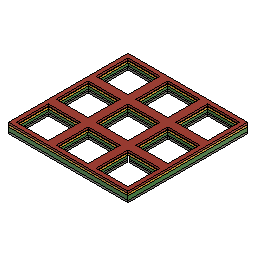
One Face (Autodesk Fusion 360 design; units mm, degrees)
Autodesk Fusion 360 part; units mm, degrees
note: some values were not read from the file. Set by a fixed rule: which sketch regions a step uses.
sketch "OldFirstLayer" plane through (0, 0, 0) normal (0, 0, 1) x (1, 0, 0)
  line L0 (-176.2126, -49.2126) -> (-176.2126, 49.2124)
  line L1 (-77.7876, 49.2124) -> (-77.7876, -49.2126)
  line L2 (-77.7876, 77.7874) -> (-176.2126, 77.7874)
  line L3 (-77.7876, 176.2124) -> (-77.7876, 77.7874)
  line L4 (-176.2126, 176.2124) -> (-77.7876, 176.2124)
  line L5 (-176.2126, -176.2126) -> (-176.2126, -77.7876)
  line L6 (-77.7876, -86.1838) -> (-77.7876, -176.2126)
  line L7 (-176.2126, 49.2124) -> (-77.7876, 49.2124)
  line L8 (-77.7876, -176.2126) -> (-176.2126, -176.2126)
  line L9 (49.2124, -82.6672) -> (49.2124, -176.2126)
  line L10 (190.4999, -190.5001) -> (190.4999, 190.4999)
  line L11 (49.2124, 176.2124) -> (49.2124, 77.7874)
  line L12 (176.2124, -176.2126) -> (77.7874, -176.2126)
  line L13 (77.7874, -49.2126) -> (77.7874, 49.2124)
  line L14 (176.2124, -49.2126) -> (77.7874, -49.2126)
  line L15 (77.7874, 49.2124) -> (170.2008, 49.2124)
  line L16 (176.2124, 176.2124) -> (176.2124, 77.7874)
  line L17 (176.2124, 49.2124) -> (176.2124, -49.2126)
  line L18 (49.2124, 49.2124) -> (49.2124, -49.2126)
  line L19 (77.7874, -77.7876) -> (176.2124, -77.7876)
  line L20 (77.7874, -176.2126) -> (77.7874, -82.6672)
  line L21 (77.7874, 176.2124) -> (176.2124, 176.2124)
  line L22 (170.2008, 77.7874) -> (77.7874, 77.7874)
  line L23 (176.2124, -77.7876) -> (176.2124, -176.2126)
  line L24 (77.7874, 77.7874) -> (77.7874, 176.2124)
  line L25 (-190.5001, 190.4999) -> (-190.5001, -190.5001)
  line L26 (-77.7876, -49.2126) -> (-176.2126, -49.2126)
  line L27 (190.4999, 190.4999) -> (-190.5001, 190.4999)
  line L28 (-49.2126, -77.7876) -> (49.2124, -77.7876)
  line L29 (-49.2126, -49.2126) -> (-49.2126, 49.2124)
  line L30 (49.2124, 77.7874) -> (-49.2126, 77.7874)
  line L31 (-49.2126, 176.2124) -> (49.2124, 176.2124)
  line L32 (-176.2126, -77.7876) -> (-77.7876, -77.7876)
  line L33 (-176.2126, 77.7874) -> (-176.2126, 176.2124)
  line L34 (-49.2126, -176.2126) -> (-49.2126, -86.1838)
  line L35 (-190.5001, -190.5001) -> (190.4999, -190.5001)
  line L36 (49.2124, -49.2126) -> (-49.2126, -49.2126)
  line L37 (49.2124, -176.2126) -> (-49.2126, -176.2126)
  line L38 (-49.2126, 77.7874) -> (-49.2126, 176.2124)
  line L39 (-190.5001, 190.4999) -> (190.4999, -190.5001) construction
  line L40 (-49.2126, 49.2124) -> (49.2124, 49.2124)
  line L41 (190.4999, 190.4999) -> (-190.5001, -190.5001) construction
  line L42 (170.2008, 77.7874) -> (170.2008, 49.2124)
  line L43 (176.2124, 77.7874) -> (176.2124, 49.2124)
  line L44 (49.2124, -82.6672) -> (77.7874, -82.6672)
  line L45 (49.2124, -77.7876) -> (77.7874, -77.7876)
  line L46 (-77.7876, -77.7876) -> (-49.2126, -77.7876)
  line L47 (-77.7876, -86.1838) -> (-77.7876, -83.82)
  line L48 (-49.2126, -86.1838) -> (-49.2126, -83.82)
  line L49 (-77.7876, -83.82) -> (-49.2126, -83.82)
  point P0 (-0.0001, -0.0001)
  point P1 (-0.0001, -0.0001)
  dimension "d57" = 381
  dimension "d58" = 381
  dimension "d59" = 98.425
  dimension "d60" = 98.425
  dimension "d61" = 28.575
  dimension "d62" = 98.425
  dimension "d63" = 98.425
  dimension "d64" = 28.575
  dimension "d65" = 98.425
  dimension "d66" = 98.425
  dimension "d67" = 28.575
  dimension "d68" = 98.425
  dimension "d69" = 98.425
  dimension "d70" = 98.425
  dimension "d71" = 98.425
  dimension "d72" = 28.575
  dimension "d73" = 98.425
  dimension "d74" = 98.425
  dimension "d75" = 28.575
  dimension "d76" = 28.575
  dimension "d77" = 98.425
  dimension "d78" = 98.425
  dimension "d80" = 28.575
  dimension "d81" = 98.425
  dimension "d82" = 98.425
  dimension "d83" = 98.425
  dimension "d84" = 98.425
  dimension "d85" = 28.575
  dimension "d86" = 28.575
  dimension "d87" = 28.575
  dimension "d88" = 28.575
  dimension "d89" = 14.2875
  dimension "d90" = 14.2875
  dimension "d91" = 14.2875
  dimension "d97" = 28.575
  dimension "d103" = 14.2875
  constraint perpendicular L25 L27
  constraint parallel L27 L35
  constraint parallel L10 L25
  constraint horizontal L27
  constraint coincident P1 L41
  constraint coincident P1 L39
  constraint coincident P1 P0
  constraint horizontal L4
  constraint vertical L3
  constraint horizontal L2
  constraint vertical L33
  constraint coincident L4.start L39
  constraint horizontal L7
  constraint vertical L1
  constraint horizontal L26
  constraint vertical L0
  constraint horizontal L32
  constraint vertical L6
  constraint horizontal L8
  constraint vertical L5
  constraint horizontal L31
  constraint vertical L11
  constraint horizontal L30
  constraint vertical L38
  constraint horizontal L21
  constraint vertical L16
  constraint horizontal L22
  constraint vertical L24
  constraint horizontal L40
  constraint vertical L18
  constraint horizontal L36
  constraint vertical L29
  constraint horizontal L15
  constraint vertical L17
  constraint horizontal L14
  constraint vertical L13
  constraint horizontal L19
  constraint vertical L23
  constraint horizontal L12
  constraint vertical L20
  constraint coincident L19.start L39
  constraint horizontal L28
  constraint vertical L9
  constraint horizontal L37
  constraint vertical L34
  constraint perpendicular L15 L42
  constraint perpendicular L20 L44
  constraint parallel L6 L47
  constraint perpendicular L46 L48
  constraint perpendicular L48 L49
  measures "d57" distance of L25.end L25.start
  measures "d58" distance of L10.end L25.start
  measures "d59" distance of L4.start L2.end
  measures "d60" distance of L4.start L3.start
  measures "d61" distance of L2 L7
  measures "d62" distance of L0.end L0.start
  measures "d63" distance of L0.end L1.start
  measures "d64" distance of L26 L32
  measures "d65" distance of L6.end L5.start
  measures "d66" distance of L6.end L32.end
  measures "d67" distance of L3 L38
  measures "d68" distance of L11.end L30.end
  measures "d69" distance of L11.end L11.start
  measures "d70" distance of L21.start L16.start
  measures "d71" distance of L16.start L16.end
  measures "d72" distance of L11 L24
  measures "d73" distance of L29.end L18.start
  measures "d74" distance of L29.end L29.start
  measures "d75" distance of L1 L29
  measures "d76" distance of L30 L40
  measures "d77" distance of L13.end L17.start
  measures "d78" distance of L13.start L13.end
  measures "d80" distance of L15 L22
  measures "d81" distance of L19.end L12.start
  measures "d82" distance of L19.start L19.end
  measures "d83" distance of L28.end L28.start
  measures "d84" distance of L34.start L28.start
  measures "d85" distance of L28 L36
  measures "d86" distance of L6 L34
  measures "d87" distance of L9 L20
  measures "d88" distance of L14 L19
  measures "d89" distance of L25 L33
  measures "d90" distance of L0 L25
  measures "d91" distance of L5 L25
  measures "d97" distance of L13 L18
  measures "d103" distance of L35 L37
sketch "ThirdLayerSketch" plane through (0, 0, 0) normal (0, 0, 1) x (1, 0, 0)
  line L0 (48.9649, -178.1983) -> (-49.4601, -178.1983)
  line L1 (-49.4601, 174.2267) -> (48.9649, 174.2267)
  line L2 (-49.4601, -79.7733) -> (48.9649, -79.7733)
  line L3 (48.9649, 47.2267) -> (48.9649, -51.1983)
  line L4 (48.9649, 174.2267) -> (48.9649, 75.8017)
  line L5 (77.5399, 174.2267) -> (175.9649, 174.2267)
  line L6 (175.9649, 174.2267) -> (175.9649, 75.8017)
  line L7 (175.9649, 47.2267) -> (175.9649, -51.1983)
  line L8 (-78.0351, -51.1983) -> (-176.4601, -51.1983)
  line L9 (175.9649, -178.1983) -> (77.5399, -178.1983)
  line L10 (48.9649, -79.7733) -> (48.9649, -178.1983)
  line L11 (175.9649, -51.1983) -> (77.5399, -51.1983)
  line L12 (-176.4601, -79.7733) -> (-78.0351, -79.7733)
  line L13 (-78.0351, -178.1983) -> (-176.4601, -178.1983)
  line L14 (175.9649, -79.7733) -> (175.9649, -178.1983)
  line L15 (77.5399, -178.1983) -> (77.5399, -79.7733)
  line L16 (77.5399, -79.7733) -> (175.9649, -79.7733)
  line L17 (-176.4601, 174.2267) -> (-78.0351, 174.2267)
  line L18 (-78.0351, 47.2267) -> (-78.0351, -51.1983)
  line L19 (-176.4601, 75.8017) -> (-176.4601, 174.2267)
  line L20 (-176.4601, -178.1983) -> (-176.4601, -79.7733)
  line L21 (77.5399, 47.2267) -> (175.9649, 47.2267)
  line L22 (77.5399, -51.1983) -> (77.5399, 47.2267)
  line L23 (-78.0351, -79.7733) -> (-78.0351, -178.1983)
  line L24 (175.9649, 75.8017) -> (77.5399, 75.8017)
  line L25 (-190.7476, 188.5142) -> (-190.7476, -192.4858)
  line L26 (190.2524, -192.4858) -> (190.2524, 188.5142)
  line L27 (77.5399, 75.8017) -> (77.5399, 174.2267)
  line L28 (-176.4601, -51.1983) -> (-176.4601, 47.2267)
  line L29 (-176.4601, 47.2267) -> (-78.0351, 47.2267)
  line L30 (-78.0351, 174.2267) -> (-78.0351, 75.8017)
  line L31 (-49.4601, 47.2267) -> (48.9649, 47.2267)
  line L32 (-78.0351, 75.8017) -> (-176.4601, 75.8017)
  line L33 (190.2524, 188.5142) -> (-190.7476, 188.5142)
  line L34 (-49.4601, 75.8017) -> (-49.4601, 174.2267)
  line L35 (48.9649, 75.8017) -> (-49.4601, 75.8017)
  line L36 (-49.4601, -51.1983) -> (-49.4601, 47.2267)
  line L37 (48.9649, -51.1983) -> (-49.4601, -51.1983)
  line L38 (-190.7476, -192.4858) -> (190.2524, -192.4858)
  line L39 (-49.4601, -178.1983) -> (-49.4601, -79.7733)
  point P0 (-0.2476, -1.9858)
  point P1 (-2.792, -21.275)
  point P2 (-0.2476, -1.9858)
  dimension "d109" = 381
  dimension "d110" = 381
  dimension "d111" = 98.425
  dimension "d112" = 98.425
  dimension "d113" = 28.575
  dimension "d114" = 98.425
  dimension "d115" = 98.425
  dimension "d116" = 28.575
  dimension "d117" = 98.425
  dimension "d118" = 98.425
  dimension "d119" = 28.575
  dimension "d120" = 98.425
  dimension "d121" = 98.425
  dimension "d122" = 98.425
  dimension "d123" = 98.425
  dimension "d124" = 28.575
  dimension "d125" = 98.425
  dimension "d126" = 98.425
  dimension "d127" = 28.575
  dimension "d128" = 28.575
  dimension "d129" = 98.425
  dimension "d130" = 98.425
  dimension "d131" = 28.575
  dimension "d132" = 98.425
  dimension "d133" = 98.425
  dimension "d134" = 98.425
  dimension "d135" = 98.425
  dimension "d136" = 28.575
  dimension "d137" = 28.575
  dimension "d138" = 28.575
  dimension "d139" = 28.575
  dimension "d140" = 14.2875
  dimension "d141" = 14.2875
  dimension "d142" = 14.2875
  dimension "d143" = 28.575
  dimension "d144" = 14.2875
  constraint perpendicular L25 L33
  constraint parallel L33 L38
  constraint parallel L25 L26
  constraint horizontal L33
  constraint coincident P2 P0
  constraint horizontal L17
  constraint vertical L30
  constraint horizontal L32
  constraint vertical L19
  constraint horizontal L29
  constraint vertical L18
  constraint horizontal L8
  constraint vertical L28
  constraint horizontal L12
  constraint vertical L23
  constraint horizontal L13
  constraint vertical L20
  constraint horizontal L1
  constraint vertical L4
  constraint horizontal L35
  constraint vertical L34
  constraint horizontal L5
  constraint vertical L6
  constraint horizontal L24
  constraint vertical L27
  constraint horizontal L31
  constraint vertical L3
  constraint horizontal L37
  constraint vertical L36
  constraint horizontal L21
  constraint vertical L7
  constraint horizontal L11
  constraint vertical L22
  constraint horizontal L16
  constraint vertical L14
  constraint horizontal L9
  constraint vertical L15
  constraint horizontal L2
  constraint vertical L10
  constraint horizontal L0
  constraint vertical L39
  measures "d109" distance of L25.start L25.end
  measures "d110" distance of L25.start L26.end
  measures "d111" distance of L17.start L19.start
  measures "d112" distance of L17.start L17.end
  measures "d113" distance of L29 L32
  measures "d114" distance of L8.end L28.end
  measures "d115" distance of L28.end L18.start
  measures "d116" distance of L8 L12
  measures "d117" distance of L13.start L13.end
  measures "d118" distance of L13.start L12.end
  measures "d119" distance of L30 L34
  measures "d120" distance of L34.start L4.end
  measures "d121" distance of L1.end L4.end
  measures "d122" distance of L5.start L5.end
  measures "d123" distance of L6.end L5.end
  measures "d124" distance of L4 L27
  measures "d125" distance of L3.start L31.start
  measures "d126" distance of L31.start L36.start
  measures "d127" distance of L18 L36
  measures "d128" distance of L31 L35
  measures "d129" distance of L21.start L7.start
  measures "d130" distance of L21.start L11.end
  measures "d131" distance of L21 L24
  measures "d132" distance of L14.start L9.start
  measures "d133" distance of L14.start L15.end
  measures "d134" distance of L2.start L2.end
  measures "d135" distance of L0.end L2.start
  measures "d136" distance of L2 L37
  measures "d137" distance of L23 L39
  measures "d138" distance of L10 L15
  measures "d139" distance of L11 L16
  measures "d140" distance of L19 L25
  measures "d141" distance of L25 L28
  measures "d142" distance of L20 L25
  measures "d143" distance of L3 L22
  measures "d144" distance of L0 L38
sketch "FourthLayerSketch" plane through (0, 0, 0) normal (0, 0, 1) x (1, 0, 0)
  line L0 (177.8, -177.8) -> (76.2, -177.8)
  line L1 (-76.2, 50.8) -> (-76.2, -50.8)
  line L2 (-50.8, -76.2) -> (50.8, -76.2)
  line L3 (-177.8, 76.2) -> (-177.8, 177.8)
  line L4 (-76.2, -177.8) -> (-177.8, -177.8)
  line L5 (-177.8, -76.2) -> (-76.2, -76.2)
  line L6 (-76.2, 76.2) -> (-177.8, 76.2)
  line L7 (-177.8, 177.8) -> (-76.2, 177.8)
  line L8 (-50.8, 177.8) -> (50.8, 177.8)
  line L9 (-76.2, 177.8) -> (-76.2, 76.2)
  line L10 (190.5, 190.5) -> (-190.5, 190.5)
  line L11 (190.5, 190.5) -> (-190.5, -190.5) construction
  line L12 (-177.8, -50.8) -> (-177.8, 50.8)
  line L13 (-50.8, 50.8) -> (50.8, 50.8)
  line L14 (-190.5, -190.5) -> (190.5, -190.5)
  line L15 (-76.2, -50.8) -> (-177.8, -50.8)
  line L16 (-50.8, -177.8) -> (-50.8, -76.2)
  line L17 (-76.2, -76.2) -> (-76.2, -177.8)
  line L18 (50.8, -50.8) -> (-50.8, -50.8)
  line L19 (50.8, 76.2) -> (-50.8, 76.2)
  line L20 (-177.8, 50.8) -> (-76.2, 50.8)
  line L21 (-50.8, 76.2) -> (-50.8, 177.8)
  line L22 (-177.8, -177.8) -> (-177.8, -76.2)
  line L23 (-190.5, 190.5) -> (-190.5, -190.5)
  line L24 (-190.5, 190.5) -> (190.5, -190.5) construction
  line L25 (50.8, -177.8) -> (-50.8, -177.8)
  line L26 (-50.8, -50.8) -> (-50.8, 50.8)
  line L27 (76.2, 50.8) -> (177.8, 50.8)
  line L28 (50.8, 50.8) -> (50.8, -50.8)
  line L29 (177.8, -76.2) -> (177.8, -177.8)
  line L30 (177.8, 50.8) -> (177.8, -50.8)
  line L31 (190.5, -190.5) -> (190.5, 190.5)
  line L32 (50.8, 177.8) -> (50.8, 76.2)
  line L33 (76.2, -76.2) -> (177.8, -76.2)
  line L34 (76.2, 177.8) -> (177.8, 177.8)
  line L35 (76.2, -50.8) -> (76.2, 50.8)
  line L36 (177.8, 177.8) -> (177.8, 76.2)
  line L37 (76.2, -177.8) -> (76.2, -76.2)
  line L38 (177.8, -50.8) -> (76.2, -50.8)
  line L39 (50.8, -76.2) -> (50.8, -177.8)
  line L40 (177.8, 76.2) -> (76.2, 76.2)
  line L41 (76.2, 76.2) -> (76.2, 177.8)
  dimension "d186" = 381
  dimension "d187" = 381
  dimension "d188" = 101.6
  dimension "d189" = 101.6
  dimension "d190" = 25.4
  dimension "d191" = 101.6
  dimension "d192" = 101.6
  dimension "d193" = 25.4
  dimension "d194" = 101.6
  dimension "d195" = 101.6
  dimension "d196" = 25.4
  dimension "d197" = 101.6
  dimension "d198" = 101.6
  dimension "d199" = 101.6
  dimension "d200" = 101.6
  dimension "d201" = 25.4
  dimension "d202" = 101.6
  dimension "d203" = 101.6
  dimension "d204" = 25.4
  dimension "d205" = 25.4
  dimension "d206" = 101.6
  dimension "d207" = 101.6
  dimension "d208" = 25.4
  dimension "d209" = 101.6
  dimension "d210" = 101.6
  dimension "d211" = 101.6
  dimension "d212" = 101.6
  dimension "d213" = 25.4
  dimension "d214" = 25.4
  dimension "d215" = 25.4
  dimension "d216" = 25.4
  dimension "d217" = 12.7
  dimension "d218" = 12.7
  dimension "d219" = 12.7
  dimension "d220" = 25.4
  dimension "d221" = 12.7
  constraint perpendicular L10 L23
  constraint parallel L10 L14
  constraint parallel L23 L31
  constraint horizontal L10
  constraint coincident origin L11
  constraint coincident origin L24
  constraint horizontal L7
  constraint vertical L9
  constraint horizontal L6
  constraint vertical L3
  constraint coincident L3.end L24
  constraint horizontal L20
  constraint vertical L1
  constraint horizontal L15
  constraint vertical L12
  constraint horizontal L5
  constraint vertical L17
  constraint horizontal L4
  constraint vertical L22
  constraint horizontal L8
  constraint vertical L32
  constraint horizontal L19
  constraint vertical L21
  constraint horizontal L34
  constraint vertical L36
  constraint horizontal L40
  constraint vertical L41
  constraint horizontal L13
  constraint vertical L28
  constraint horizontal L18
  constraint vertical L26
  constraint horizontal L27
  constraint vertical L30
  constraint horizontal L38
  constraint vertical L35
  constraint horizontal L33
  constraint vertical L29
  constraint horizontal L0
  constraint vertical L37
  constraint coincident L33.start L24
  constraint horizontal L2
  constraint vertical L39
  constraint horizontal L25
  constraint vertical L16
  measures "d186" distance of L10.end L11.end
  measures "d187" distance of L10.end L10.start
  measures "d188" distance of L3.end L3.start
  measures "d189" distance of L3.end L7.end
  measures "d190" distance of L6 L20
  measures "d191" distance of L12.start L12.end
  measures "d192" distance of L1.start L12.end
  measures "d193" distance of L5 L15
  measures "d194" distance of L4.start L4.end
  measures "d195" distance of L5.end L4.start
  measures "d196" distance of L9 L21
  measures "d197" distance of L19.start L19.end
  measures "d198" distance of L8.end L19.start
  measures "d199" distance of L34.end L34.start
  measures "d200" distance of L36.end L34.end
  measures "d201" distance of L32 L41
  measures "d202" distance of L13.start L13.end
  measures "d203" distance of L13.start L18.end
  measures "d204" distance of L1 L26
  measures "d205" distance of L13 L19
  measures "d206" distance of L27.start L27.end
  measures "d207" distance of L35.start L27.start
  measures "d208" distance of L27 L40
  measures "d209" distance of L29.start L0.start
  measures "d210" distance of L29.start L33.start
  measures "d211" distance of L2.end L2.start
  measures "d212" distance of L16.start L2.start
  measures "d213" distance of L2 L18
  measures "d214" distance of L16 L17
  measures "d215" distance of L37 L39
  measures "d216" distance of L33 L38
  measures "d217" distance of L3 L23
  measures "d218" distance of L12 L23
  measures "d219" distance of L22 L23
  measures "d220" distance of L28 L35
  measures "d221" distance of L14 L25
sketch "SecondLayerSketch" plane through (0, 0, 0) normal (0, 0, 1) x (1, 0, 0)
  line L0 (-73.66, -79.2817) -> (-73.66, -181.6847)
  line L1 (-73.66, 180.2653) -> (-73.66, 79.042)
  line L2 (189.865, 189.8689) -> (-191.135, 189.8689)
  line L3 (-54.61, -46.0564) -> (-54.61, 53.3439)
  line L4 (-79.9355, -54.6847) -> (-181.61, -54.6847)
  line L5 (-76.9875, 72.3153) -> (-181.61, 72.3153)
  line L6 (-181.61, -73.7347) -> (-80.5215, -73.7347)
  line L7 (-47.546, -73.6561) -> (53.2937, -73.6561)
  line L8 (-54.61, 81.5617) -> (-54.61, 180.9702)
  line L9 (47.3923, -54.6061) -> (-45.4633, -54.6061)
  line L10 (-191.135, 189.8689) -> (-191.135, -191.1311)
  line L11 (53.34, -82.5688) -> (53.34, -181.6061)
  line L12 (-181.61, 180.2653) -> (-73.66, 180.2653)
  line L13 (72.39, 180.9702) -> (180.34, 180.9702)
  line L14 (-181.61, -181.6847) -> (-181.61, -73.7347)
  line L15 (-181.61, -54.6847) -> (-181.61, 53.2653)
  line L16 (-73.66, -181.6847) -> (-181.61, -181.6847)
  line L17 (180.34, 53.9702) -> (180.34, -53.9797)
  line L18 (53.34, 49.1036) -> (53.34, -43.5643)
  line L19 (-73.66, 44.9474) -> (-73.66, -52.5872)
  line L20 (-181.61, 72.3153) -> (-181.61, 180.2653)
  line L21 (-54.61, -181.6061) -> (-54.61, -73.6561)
  line L22 (78.7065, 53.9703) -> (170.0179, 53.9703)
  line L23 (180.34, -180.9797) -> (72.39, -180.9797)
  line L24 (72.39, 92.2139) -> (72.39, 180.9702)
  line L25 (180.34, -73.0297) -> (180.34, -180.9797)
  line L26 (-46.1443, 53.3439) -> (37.3349, 53.3439)
  line L27 (72.39, -180.9797) -> (72.39, -77.2123)
  line L28 (53.34, 180.9702) -> (53.34, 79.0294)
  line L29 (180.34, -53.9797) -> (81.8994, -53.9797)
  line L30 (189.865, -191.1311) -> (189.865, 189.8689)
  line L31 (53.34, -181.6061) -> (-54.61, -181.6061)
  line L32 (-191.135, -191.1311) -> (189.865, -191.1311)
  line L33 (80.8298, -73.0297) -> (180.34, -73.0297)
  line L34 (72.39, -41.8895) -> (72.39, 53.8895)
  line L35 (180.34, 180.9702) -> (180.34, 73.0202)
  line L36 (-54.61, 180.9702) -> (53.34, 180.9702)
  line L37 (170.0179, 73.0203) -> (77.4412, 73.0203)
  line L38 (52.7048, 73.0202) -> (-54.61, 73.0202)
  line L39 (65.0277, -69.85) -> (53.34, -82.5688)
  line L40 (61.0314, -65.9185) -> (53.2937, -73.6561)
  line L41 (73.75, -65.95) -> (80.8298, -73.0297)
  line L42 (-73.66, -52.5872) -> (-66.37, -59.8172)
  line L43 (-80.5215, -73.7347) -> (-70.7062, -63.8379)
  line L44 (-79.9355, -54.6847) -> (-70.7062, -63.8379)
  line L45 (-73.66, -79.2817) -> (-60.4068, -65.9185)
  line L46 (62.5235, 48.3233) -> (62.9915, -60.96)
  line L47 (68.58, 48.7134) -> (68.58, -49.4987)
  line L48 (-59.8809, -60.96) -> (62.9915, -60.96)
  line L49 (-60.4068, -65.9185) -> (61.0314, -65.9185)
  line L50 (53.34, -43.5643) -> (53.34, -54.6061)
  line L51 (53.34, -54.6061) -> (47.3923, -54.6061)
  line L52 (-54.61, -46.0564) -> (-54.61, -54.6061)
  line L53 (-54.61, -54.6061) -> (-45.4633, -54.6061)
  line L54 (72.39, -41.8895) -> (72.39, -53.9797)
  line L55 (72.39, -53.9797) -> (81.8994, -53.9797)
  line L56 (68.58, -49.4987) -> (68.58, -60.7799)
  line L57 (68.58, -60.7799) -> (73.75, -65.95)
  line L58 (-47.546, -73.6561) -> (-54.61, -73.6561)
  line L59 (-54.61, 81.5617) -> (-54.61, 73.0202)
  line L60 (-46.1443, 53.3439) -> (-54.61, 53.3439)
  line L61 (-73.66, 44.9474) -> (-73.66, 53.2653)
  line L62 (-66.37, -59.8172) -> (-66.37, 64.2542)
  line L63 (-59.8809, -59.3014) -> (-59.8809, 67.2074)
  line L64 (-59.8809, 67.2074) -> (-73.66, 79.042)
  line L65 (-76.9875, 72.3153) -> (-66.37, 64.2542)
  line L66 (170.0179, 73.0203) -> (180.34, 73.0202)
  line L67 (170.0179, 53.9703) -> (180.34, 53.9702)
  line L68 (62.5235, 48.3233) -> (62.4814, 58.1673)
  line L69 (68.58, 48.7134) -> (68.58, 57.5922)
  line L70 (62.4814, 58.1673) -> (53.34, 49.1036)
  line L71 (72.39, 92.2139) -> (72.39, 73.8255)
  line L72 (37.3349, 53.3439) -> (51.9517, 53.3439)
  line L73 (51.9517, 53.3439) -> (62.2905, 63.7046)
  line L74 (65.5482, 66.9691) -> (72.39, 73.8255)
  line L75 (52.7048, 73.0202) -> (62.2905, 63.7046)
  line L76 (68.58, 57.5922) -> (72.39, 53.8895)
  line L77 (77.4412, 73.0203) -> (68.3501, 64.2012)
  line L78 (53.34, 79.0294) -> (65.5482, 66.9691)
  line L79 (68.3501, 64.2012) -> (78.7065, 53.9703)
  line L80 (-59.8809, -59.3014) -> (-59.8809, -60.96)
  line L81 (72.39, -77.2123) -> (65.0277, -69.85)
  line L82 (-181.61, 53.2653) -> (-73.66, 53.2653)
  point P0 (0.0009, -0.0048)
  point P1 (-36.3144, 12.7463)
  point P2 (-36.3144, 12.7463)
  point P3 (-36.3144, 12.7463)
  point P4 (0.0009, -0.0048)
  dimension "d233" = 381
  dimension "d234" = 381
  dimension "d235" = 107.95
  dimension "d236" = 107.95
  dimension "d237" = 19.05
  dimension "d238" = 107.95
  dimension "d240" = 19.05
  dimension "d241" = 107.95
  dimension "d243" = 19.05
  dimension "d246" = 107.95
  dimension "d247" = 107.95
  dimension "d248" = 19.05
  dimension "d251" = 19.05
  dimension "d255" = 19.05
  dimension "d256" = 107.95
  dimension "d260" = 19.05
  dimension "d261" = 19.05
  dimension "d262" = 19.05
  dimension "d263" = 19.05
  dimension "d264" = 9.525
  dimension "d265" = 9.525
  dimension "d266" = 9.525
  dimension "d267" = 19.05
  dimension "d268" = 9.525
  dimension "d325" = 107.95
  dimension "d326" = 107.95
  dimension "d327" = 107.95
  dimension "d328" = 107.95
  dimension "d329" = 107.95
  dimension "d330" = 107.95
  dimension "d331" = 107.95
  dimension "d332" = 107.95
  dimension "d333" = 107.95
  dimension "d334" = 107.95
  dimension "d335" = 107.95
  constraint perpendicular L2 L10
  constraint parallel L2 L32
  constraint parallel L10 L30
  constraint horizontal L2
  constraint coincident P4 P0
  constraint horizontal L12
  constraint vertical L1
  constraint horizontal L5
  constraint vertical L20
  constraint horizontal L82
  constraint vertical L19
  constraint horizontal L4
  constraint vertical L15
  constraint horizontal L6
  constraint vertical L0
  constraint horizontal L16
  constraint vertical L14
  constraint horizontal L36
  constraint vertical L28
  constraint vertical L8
  constraint horizontal L13
  constraint vertical L35
  constraint horizontal L37
  constraint vertical L24
  constraint horizontal L26
  constraint vertical L18
  constraint horizontal L9
  constraint vertical L3
  constraint horizontal L22
  constraint vertical L17
  constraint horizontal L29
  constraint vertical L34
  constraint horizontal L33
  constraint vertical L25
  constraint horizontal L23
  constraint vertical L27
  constraint horizontal L7
  constraint vertical L11
  constraint horizontal L31
  constraint vertical L21
  constraint parallel L42 L44
  constraint perpendicular L42 L43
  constraint parallel L43 L45
  constraint parallel L7 L48
  constraint horizontal L49
  constraint perpendicular L18 L51
  constraint parallel L3 L52
  constraint perpendicular L3 L53
  constraint parallel L34 L54
  constraint perpendicular L54 L55
  constraint parallel L47 L56
  constraint parallel L7 L58
  constraint parallel L8 L59
  constraint parallel L26 L60
  constraint vertical L61
  constraint vertical L62
  constraint parallel L62 L63
  constraint parallel L66 L67
  constraint parallel L46 L68
  constraint parallel L47 L69
  constraint parallel L28 L71
  constraint parallel L26 L72
  constraint vertical L69
  constraint horizontal L38
  constraint coincident L69.end L75
  constraint collinear L73 L74
  constraint collinear L75 L76
  constraint coincident L77.end L78
  constraint collinear L78 L79
  constraint parallel L63 L80
  constraint perpendicular L40 L81
  measures "d233" distance of L10.end L2.end
  measures "d234" distance of L2.start L2.end
  measures "d235" distance of L12.start L5.end
  measures "d236" distance of L1.start L12.start
  measures "d237" distance of L5 L82
  measures "d238" distance of L4.end L15.end
  measures "d240" distance of L4 L6
  measures "d241" distance of L14.start L0.end
  measures "d243" distance of L1 L8
  measures "d246" distance of L13.end L13.start
  measures "d247" distance of L13.end L35.end
  measures "d248" distance of L24 L28
  measures "d251" distance of L3 L19
  measures "d255" distance of L22 L37
  measures "d256" distance of L25.start L23.start
  measures "d260" distance of L7 L9
  measures "d261" distance of L0 L21
  measures "d262" distance of L11 L27
  measures "d263" distance of L29 L33
  measures "d264" distance of L10 L20
  measures "d265" distance of L10 L15
  measures "d266" distance of L10 L14
  measures "d267" distance of L18 L34
  measures "d268" distance of L31 L32
  measures "d325" distance of L11 L21
  measures "d326" distance of L6 L16
  measures "d327" distance of L25 L27
  measures "d328" distance of L22 L29
  measures "d329" distance of L17 L34
  measures "d330" distance of L9 L26
  measures "d331" distance of L3 L18
  measures "d332" distance of L36 L38
  measures "d333" distance of L8 L28
  measures "d334" distance of L15 L19
  measures "d335" distance of L7 L31
extrude "Extrude9" add sketch "FourthLayerSketch" along normal blind 6.35 makes body 1
move_body "Move14" bodies 1 to x (1, 0, 0) y (0, 1, 0) z (0, 0, 1) at (0, 0, 25.4)
extrude "Extrude11" add sketch "SecondLayerSketch" along normal blind 12.7 separate body makes body 2
extrude "Extrude12" add sketch "ThirdLayerSketch" along normal blind 6.35 separate body makes body 3
move_body "Move15" bodies 3 to x (1, 0, 0) y (0, 1, 0) z (0, 0, 1) at (0, 0, 19.05)
move_body "Move16" bodies 2 to x (1, 0, 0) y (0, 1, 0) z (0, 0, 1) at (0, 0, 6.35)
move_body "Align1" bodies 2 to x (1, 0, 0) y (0, 1, 0) z (0, 0, 1) at (0, 0, 0)
move_body "Align2" bodies 2 to x (1, 0, 0) y (0, 1, 0) z (0, 0, 1) at (0, 0.631, 0)
move_body "Align3" bodies 2 to x (1, 0, 0) y (0, 1, 0) z (0, 0, 1) at (0.6349, 0, 0)
move_body "Align4" bodies 3 to x (1, 0, 0) y (0, 1, 0) z (0, 0, 1) at (0, 0, 0)
move_body "Align5" bodies 3 to x (1, 0, 0) y (0, 1, 0) z (0, 0, 1) at (0, 1.9857, 0)
move_body "Align6" bodies 3 to x (1, 0, 0) y (0, 1, 0) z (0, 0, 1) at (0.2475, 0, 0)
move_body "Align7" bodies 1 to x (1, 0, 0) y (0, 1, 0) z (0, 0, 1) at (0, 0, 0)
move_body "Align8" bodies 1 to x (1, 0, 0) y (0, 1, 0) z (0, 0, 1) at (-0.0001, 0, 0)
move_body "Align9" bodies 1 to x (1, 0, 0) y (0, 1, 0) z (0, 0, 1) at (0, -0.0001, 0)
sketch "FirstLayerSketch" plane through (0, 0, 0) normal (0, 0, 1) x (1, 0, 0)
  line L0 (48.5648, -89.3191) -> (48.5648, -176.8409)
  line L1 (77.1398, -49.9169) -> (77.1398, 48.5841)
  line L2 (38.2406, 48.5841) -> (47.3405, 48.5841)
  line L3 (175.5648, 48.5841) -> (175.5648, -49.8409)
  line L4 (48.298, -49.8409) -> (-49.8602, -49.8409)
  line L5 (48.5648, 44.606) -> (48.5648, -49.8409)
  line L6 (175.5648, -176.8409) -> (77.1398, -176.8409)
  line L7 (-49.8602, -176.8409) -> (-49.8602, -78.4159)
  line L8 (-176.8602, -176.8409) -> (-176.8602, -78.4159)
  line L9 (48.5648, -176.8409) -> (-49.8602, -176.8409)
  line L10 (77.1398, -176.8409) -> (77.1398, -82.0046)
  line L11 (170.8663, 48.5841) -> (175.5648, 48.5841)
  line L12 (48.5648, -49.8409) -> (48.298, -49.8409)
  line L13 (77.1398, -49.9169) -> (82.2599, -49.8409)
  line L14 (175.5648, -49.8409) -> (82.2599, -49.8409)
  line L15 (-45.2386, 48.5841) -> (38.2406, 48.5841)
  line L16 (-78.4352, -83.6713) -> (-78.4352, -176.8409)
  line L17 (-49.8602, -78.4159) -> (48.6937, -78.4159)
  line L18 (175.5648, -78.4159) -> (175.5648, -176.8409)
  line L19 (86.3918, -78.4159) -> (175.5648, -78.4159)
  line L20 (-191.1477, -191.1284) -> (189.8523, -191.1284)
  line L21 (77.1398, 175.5841) -> (175.5648, 175.5841)
  line L22 (-191.1477, 189.8716) -> (-191.1477, -191.1284)
  line L23 (77.1398, 78.803) -> (77.1398, 175.5841)
  line L24 (175.5648, 175.5841) -> (175.5648, 77.1591)
  line L25 (163.7334, 77.1591) -> (175.5648, 77.1591)
  line L26 (163.7334, 77.1591) -> (81.8586, 77.1591)
  line L27 (-78.4352, 175.5841) -> (-78.4352, 82.9985)
  line L28 (-49.8602, -49.8409) -> (-49.8602, 48.5841)
  line L29 (189.8523, -191.1284) -> (189.8523, 189.8716)
  line L30 (-83.8454, 77.1591) -> (-176.8602, 77.1591)
  line L31 (-176.8602, 77.1591) -> (-176.8602, 175.5841)
  line L32 (-176.8602, 175.5841) -> (-78.4352, 175.5841)
  line L33 (-45.2386, 48.5841) -> (-49.8602, 48.5841)
  line L34 (189.8523, 189.8716) -> (-191.1477, 189.8716)
  line L35 (-176.8602, -78.4159) -> (-85.3493, -78.4159)
  line L36 (-176.8602, -176.8409) -> (-78.4352, -176.8409)
  line L37 (48.5847, -87.639) -> (48.5648, -89.3191)
  line L38 (-176.8602, 48.5841) -> (-78.4352, 48.5841)
  line L39 (-78.4352, 48.5841) -> (-78.4352, -48.3516)
  line L40 (-85.6124, -49.8409) -> (-176.8602, -49.8409)
  line L41 (-176.8602, -49.8409) -> (-176.8602, 48.5841)
  line L42 (-49.8602, 175.5841) -> (48.5648, 175.5841)
  line L43 (48.5648, 175.5841) -> (48.5648, 83.5435)
  line L44 (47.8056, 77.1591) -> (-49.8602, 77.1591)
  line L45 (-49.8602, 77.1591) -> (-49.8602, 175.5841)
  line L46 (77.1398, 48.5841) -> (77.9225, 48.5841)
  line L47 (83.9665, 48.5841) -> (170.8663, 48.5841)
  line L48 (47.8056, 77.1591) -> (62.123, 63.5747)
  line L49 (65.0879, 60.7616) -> (77.9225, 48.5841)
  line L50 (77.1398, 78.803) -> (65.4104, 66.9084)
  line L51 (62.123, 63.5747) -> (47.3405, 48.5841)
  line L52 (81.8586, 77.1591) -> (68.3777, 63.9781)
  line L53 (65.0879, 60.7616) -> (48.5648, 44.606)
  line L54 (48.5648, 83.5435) -> (65.4104, 66.9084)
  line L55 (68.3777, 63.9781) -> (83.9665, 48.5841)
  line L56 (62.4803, 58.212) -> (62.4803, -60.96)
  line L57 (68.5827, 57.4457) -> (68.5827, -60.96)
  line L58 (68.5827, -60.96) -> (86.3918, -78.4159)
  line L59 (65.024, -69.85) -> (77.1398, -82.0046)
  line L60 (65.024, -69.85) -> (48.5847, -87.639)
  line L61 (60.96, -66.04) -> (48.6937, -78.4159)
  line L62 (60.96, -66.04) -> (-60.96, -66.04)
  line L63 (-60.96, -66.04) -> (-78.4352, -83.6713)
  line L64 (62.4803, -60.96) -> (-59.69, -60.96)
  line L65 (-59.69, -60.96) -> (-59.944, 67.31)
  line L66 (-59.944, 67.31) -> (-78.4352, 82.9985)
  line L67 (-85.3493, -78.4159) -> (-70.6924, -63.7617)
  line L68 (-70.6924, -63.7617) -> (-85.6124, -49.8409)
  line L69 (-78.4352, -48.3516) -> (-66.421, -59.69)
  line L70 (-66.421, -59.69) -> (-66.421, 63.5)
  line L71 (-66.421, 63.5) -> (-83.8454, 77.1591)
  point P0 (0.9066, -11.0178)
  point P1 (0.9066, -11.0178)
  dimension "d284" = 381
  dimension "d285" = 381
  dimension "d286" = 98.425
  dimension "d287" = 98.425
  dimension "d293" = 98.425
  dimension "d294" = 98.425
  dimension "d297" = 28.575
  dimension "d298" = 98.425
  dimension "d299" = 28.575
  dimension "d300" = 28.575
  dimension "d301" = 28.575
  dimension "d302" = 28.575
  dimension "d303" = 14.2875
  dimension "d305" = 14.2875
  dimension "d306" = 28.575
  dimension "d307" = 14.2875
  dimension "d308" = 98.425
  dimension "d309" = 98.425
  dimension "d310" = 98.425
  dimension "d311" = 98.425
  dimension "d313" = 98.425
  dimension "d314" = 98.425
  dimension "d316" = 98.425
  dimension "d317" = 98.425
  dimension "d321" = 14.2875
  dimension "d322" = 14.2875
  dimension "d336" = 98.425
  dimension "d339" = 14.2875
  dimension "d340" = 98.425
  dimension "d341" = 98.425
  dimension "d342" = 28.575
  dimension "d343" = 28.575
  dimension "d344" = 28.575
  dimension "d345" = 98.425
  dimension "d346" = 98.425
  dimension "d348" = 28.575
  dimension "d349" = 28.575
  dimension "d350" = 14.2875
  dimension "d351" = 14.2875
  constraint perpendicular L22 L34
  constraint parallel L20 L34
  constraint parallel L22 L29
  constraint horizontal L34
  constraint coincident P1 P0
  constraint horizontal L32
  constraint vertical L27
  constraint horizontal L30
  constraint vertical L31
  constraint vertical L16
  constraint vertical L8
  constraint horizontal L21
  constraint vertical L24
  constraint horizontal L26
  constraint vertical L23
  constraint horizontal L15
  constraint vertical L5
  constraint horizontal L4
  constraint vertical L28
  constraint horizontal L46
  constraint vertical L3
  constraint horizontal L14
  constraint vertical L1
  constraint horizontal L19
  constraint vertical L18
  constraint horizontal L6
  constraint vertical L10
  constraint horizontal L17
  constraint vertical L0
  constraint horizontal L9
  constraint vertical L7
  constraint perpendicular L5 L12
  constraint parallel L15 L33
  constraint parallel L11 L25
  constraint parallel L2 L15
  constraint perpendicular L16 L35
  constraint perpendicular L16 L36
  constraint horizontal L38
  constraint vertical L39
  constraint horizontal L40
  constraint vertical L41
  constraint horizontal L42
  constraint vertical L43
  constraint horizontal L44
  constraint vertical L45
  constraint coincident L47.start L46
  constraint collinear L46 L47
  constraint coincident L48.end L50
  constraint coincident L49.start L52
  constraint collinear L48 L49
  constraint collinear L50 L51
  constraint coincident L52.end L54
  constraint collinear L52 L53
  constraint collinear L54 L55
  constraint coincident L53 L56.start
  constraint vertical L56
  constraint coincident L49 L57.start
  constraint vertical L57
  constraint perpendicular L39 L62
  constraint parallel L61 L63
  constraint perpendicular L56 L64
  constraint parallel L39 L70
  measures "d284" distance of L22.start L20.start
  measures "d285" distance of L22.start L29.end
  measures "d286" distance of L31.end L30.end
  measures "d287" distance of L31.end L27.start
  measures "d293" distance of L21.start L21.end
  measures "d294" distance of L21.end L24.end
  measures "d297" distance of L26 L46
  measures "d298" distance of L18.start L6.start
  measures "d299" distance of L4 L17
  measures "d300" distance of L7 L16
  measures "d301" distance of L0 L10
  measures "d302" distance of L14 L19
  measures "d303" distance of L22 L31
  measures "d305" distance of L8 L22
  measures "d306" distance of L1 L5
  measures "d307" distance of L9 L20
  measures "d308" distance of L10 L18
  measures "d309" distance of L9 L17
  measures "d310" distance of L0 L7
  measures "d311" distance of L35 L36
  measures "d313" distance of L5 L28
  measures "d314" distance of L4 L15
  measures "d316" distance of L14 L46
  measures "d317" distance of L1 L3
  measures "d321" distance of L24 L29
  measures "d322" distance of L6 L20
  measures "d336" distance of L8 L16
  measures "d339" distance of L22 L41
  measures "d340" distance of L38 L40
  measures "d341" distance of L39 L41
  measures "d342" distance of L30 L38
  measures "d343" distance of L35 L40
  measures "d344" distance of L28 L39
  measures "d345" distance of L43 L45
  measures "d346" distance of L42 L44
  measures "d348" distance of L27 L45
  measures "d349" distance of L15 L44
  measures "d350" distance of L20 L36
  measures "d351" distance of L21 L34
move_body "Align10" bodies 2 to x (1, 0, 0) y (0, 1, 0) z (0, 0, 1) at (0, -0.6283, 0)
move_body "Align11" bodies 2 to x (1, 0, 0) y (0, 1, 0) z (0, 0, 1) at (-0.6476, 0, 0)
extrude "Extrude14" add sketch "FirstLayerSketch" along normal blind 6.35 separate body makes body 4
move_body "Align12" bodies 2 to x (1, 0, 0) y (0, 1, 0) z (0, 0, 1) at (0, 0, 0)
move_body "Align13" bodies 2 to x (1, 0, 0) y (0, 1, 0) z (0, 0, 1) at (0, 0, 0)
move_body "Align14" bodies 3 to x (1, 0, 0) y (0, 1, 0) z (0, 0, 1) at (0, -0.6283, 0)
move_body "Align15" bodies 3 to x (1, 0, 0) y (0, 1, 0) z (0, 0, 1) at (-0.6476, 0, 0)
move_body "Align16" bodies 1 to x (1, 0, 0) y (0, 1, 0) z (0, 0, 1) at (0, -0.6283, 0)
move_body "Align17" bodies 1 to x (1, 0, 0) y (0, 1, 0) z (0, 0, 1) at (-0.6476, 0, 0)
move_body "Move17" bodies 2 4 to x (0, 1, 0) y (-1, 0, 0) z (0, 0, 1) at (-78.319, 78.5515, 0)
move_body "Align18" bodies 3 to x (1, 0, 0) y (0, 1, 0) z (0, 0, 1) at (0, 78.5321, 0)
move_body "Align19" bodies 3 to x (1, 0, 0) y (0, 1, 0) z (0, 0, 1) at (-77.0429, 0, 0)
move_body "Align20" bodies 1 to x (1, 0, 0) y (0, 1, 0) z (0, 0, 1) at (-77.0429, 0, 0)
move_body "Align21" bodies 1 to x (1, 0, 0) y (0, 1, 0) z (0, 0, 1) at (0, 78.5321, 0)
move_body "Move18" bodies 2 4 to x (-1, 0, 0) y (0, -0.999848, -0.017452) z (0, -0.017452, 0.999848) at (-536.3811, -225.0645, -1.9641)
move_body "Move19" bodies 2 4 to x (1, 0, 0) y (0, -1, 0) z (0, 0, -1) at (0, -507.6136, 1.4194)
move_body "Move20" bodies 2 4 to x (0, 1, 0) y (-1, 0, 0) z (0, 0, 1) at (-1044.208, 254.1732, 0)
move_body "Move21" bodies 2 4 to x (1, 0, 0) y (0, 1, 0) z (0, 0, 1) at (-1.951, -0.6652, 30.2569)
move_body "Move22" bodies 2 4 to x (0.999848, 0, 0.017452) y (0, 1, 0) z (-0.017452, 0, 0.999848) at (0.0632, 0, 18.0181)
move_body "Move23" bodies 4 to x (1, 0, 0) y (0, 1, 0) z (0, 0, 1) at (0, 0, -12.7)
move_body "Move24" bodies 2 to x (1, 0, 0) y (0, 1, 0) z (0, 0, 1) at (0, 0, 6.35)
move_body "Move25" bodies 4 2 to x (-1, 0, 0) y (0, -1, 0) z (0, 0, 1) at (-1683.8425, -518.3151, 0)
move_body "Align22" bodies 2 to x (1, 0, 0) y (0, 1, 0) z (0, 0, 1) at (0, 5.3889, 0)
move_body "Align23" bodies 3 to x (-0.702783, 0.711404, 0) y (-0.711404, -0.702783, 0) z (0, 0, 1) at (-906.7744, -286.2414, 19.2766)
move_body "Align24" bodies 3 to x (0.711404, -0.702783, 0) y (0.702783, 0.711404, 0) z (0, 0, 1) at (205.4143, -663.6855, 0)
move_body "Align25" bodies 3 to x (1, 0, 0) y (0, 1, 0) z (0, 0, 1) at (-123.1831, 0, 0)
move_body "Align26" bodies 2 to x (1, 0, 0) y (0, 1, 0) z (0, 0, 1) at (0, -5.3889, 0)
move_body "Align27" bodies 2 to x (1, 0, 0) y (0, 1, 0) z (0, 0, 1) at (0, 0, 0)
move_body "Align28" bodies 3 to x (1, 0, 0) y (0, 1, 0) z (0, 0, 1) at (0, -5.3889, 0)
move_body "Align29" bodies 1 to x (-1, 0, 0) y (0, 1, 0) z (0, 0, -1) at (-1073.5993, -291.0238, 70.0766)
move_body "Align30" bodies 1 to x (1, 0, 0) y (0, 1, 0) z (0, 0, 1) at (0, 0, 6.35)
move_body "Align31" bodies 1 to x (1, 0, 0) y (0, 1, 0) z (0, 0, 1) at (0, -100.0125, 0)
move_body "Align32" bodies 1 to x (1, 0, 0) y (0, 1, 0) z (0, 0, 1) at (153.9875, 0, 0)
extrude "Extrude2" [suppressed]
equation "SecondLayerCube = 15 in"
equation "SecondLayerSquare = 4.25 in"
equation "SecondLayerIndent = 0.75 in"
equation "SecondLayerDepth = 0.5 in"
equation "SecondLayerSide = ( SecondLayerCube - ( ( 3 * SecondLayerSquare ) + ( 2 * SecondLayerIndent ) ) ) / 2"
equation "d57 = FirstLayerCube"
equation "d58 = FirstLayerCube"
equation "d59 = FirstLayerSquare"
equation "d60 = FirstLayerSquare"
equation "d61 = FirstLayerIndent"
equation "d62 = FirstLayerSquare"
equation "d63 = FirstLayerSquare"
equation "d64 = FirstLayerIndent"
equation "d65 = FirstLayerSquare"
equation "d66 = FirstLayerSquare"
equation "d67 = FirstLayerIndent"
equation "d68 = FirstLayerSquare"
equation "d69 = FirstLayerSquare"
equation "d70 = FirstLayerSquare"
equation "d71 = FirstLayerSquare"
equation "d72 = FirstLayerIndent"
equation "d73 = FirstLayerSquare"
equation "d74 = FirstLayerSquare"
equation "d75 = FirstLayerIndent"
equation "d76 = FirstLayerIndent"
equation "d77 = FirstLayerSquare"
equation "d78 = FirstLayerSquare"
equation "d80 = FirstLayerIndent"
equation "d81 = FirstLayerSquare"
equation "d82 = FirstLayerSquare"
equation "d83 = FirstLayerSquare"
equation "d84 = FirstLayerSquare"
equation "d85 = FirstLayerIndent"
equation "d86 = FirstLayerIndent"
equation "d87 = FirstLayerIndent"
equation "d88 = FirstLayerIndent"
equation "d89 = FirstLayerSide"
equation "d90 = FirstLayerSide"
equation "d91 = FirstLayerSide"
equation "FirstLayerCube = 15 in"
equation "FirstLayerSquare = 3.875 in"
equation "FirstLayerIndent = 1.125 in"
equation "FirstLayerDepth = 0.25 in"
equation "FirstLayerSide = ( FirstLayerCube - ( ( 3 * FirstLayerSquare ) + ( 2 * FirstLayerIndent ) ) ) / 2"
equation "d97 = FirstLayerIndent"
equation "d99 = FirstLayerDepth"
equation "d103 = FirstLayerSide"
equation "ThirdLayerCube = 15 in"
equation "ThirdLayerSquare = 3.875 in"
equation "ThirdLayerIndent = 1.125 in"
equation "ThirdLayerDepth = 0.25 in"
equation "ThirdLayerSide = ( ThirdLayerCube - ( ( 3 * ThirdLayerSquare ) + ( 2 * ThirdLayerIndent ) ) ) / 2"
equation "d109 = ThirdLayerCube"
equation "d110 = ThirdLayerCube"
equation "d111 = ThirdLayerSquare"
equation "d112 = ThirdLayerSquare"
equation "d113 = ThirdLayerIndent"
equation "d114 = ThirdLayerSquare"
equation "d115 = ThirdLayerSquare"
equation "d116 = ThirdLayerIndent"
equation "d117 = ThirdLayerSquare"
equation "d118 = ThirdLayerSquare"
equation "d119 = ThirdLayerIndent"
equation "d120 = ThirdLayerSquare"
equation "d121 = ThirdLayerSquare"
equation "d122 = ThirdLayerSquare"
equation "d123 = ThirdLayerSquare"
equation "d124 = ThirdLayerIndent"
equation "d125 = ThirdLayerSquare"
equation "d126 = ThirdLayerSquare"
equation "d127 = ThirdLayerIndent"
equation "d128 = ThirdLayerIndent"
equation "d129 = ThirdLayerSquare"
equation "d130 = ThirdLayerSquare"
equation "d131 = ThirdLayerIndent"
equation "d132 = ThirdLayerSquare"
equation "d133 = ThirdLayerSquare"
equation "d134 = ThirdLayerSquare"
equation "d135 = ThirdLayerSquare"
equation "d136 = ThirdLayerIndent"
equation "d137 = ThirdLayerIndent"
equation "d138 = ThirdLayerIndent"
equation "d139 = ThirdLayerIndent"
equation "d140 = ThirdLayerSide"
equation "d141 = ThirdLayerSide"
equation "d142 = ThirdLayerSide"
equation "d143 = ThirdLayerIndent"
equation "d144 = ThirdLayerSide"
equation "d186 = FourthLayerCube"
equation "d187 = FourthLayerCube"
equation "d188 = FourthLayerSquare"
equation "d189 = FourthLayerSquare"
equation "d190 = FourthLayerIndent"
equation "d191 = FourthLayerSquare"
equation "d192 = FourthLayerSquare"
equation "d193 = FourthLayerIndent"
equation "d194 = FourthLayerSquare"
equation "d195 = FourthLayerSquare"
equation "d196 = FourthLayerIndent"
equation "d197 = FourthLayerSquare"
equation "d198 = FourthLayerSquare"
equation "d199 = FourthLayerSquare"
equation "d200 = FourthLayerSquare"
equation "d201 = FourthLayerIndent"
equation "d202 = FourthLayerSquare"
equation "d203 = FourthLayerSquare"
equation "d204 = FourthLayerIndent"
equation "d205 = FourthLayerIndent"
equation "d206 = FourthLayerSquare"
equation "d207 = FourthLayerSquare"
equation "d208 = FourthLayerIndent"
equation "d209 = FourthLayerSquare"
equation "d210 = FourthLayerSquare"
equation "d211 = FourthLayerSquare"
equation "d212 = FourthLayerSquare"
equation "d213 = FourthLayerIndent"
equation "d214 = FourthLayerIndent"
equation "d215 = FourthLayerIndent"
equation "d216 = FourthLayerIndent"
equation "d217 = FourthLayerSide"
equation "d218 = FourthLayerSide"
equation "d219 = FourthLayerSide"
equation "d220 = FourthLayerIndent"
equation "d221 = FourthLayerSide"
equation "FourthLayerCube = 15 in"
equation "FourthLayerSquare = 4 in"
equation "FourthLayerIndent = 1 in"
equation "FourthLayerDepth = 0.25 in"
equation "FourthLayerSide = ( FourthLayerCube - ( ( 3 * FourthLayerSquare ) + ( 2 * FourthLayerIndent ) ) ) / 2"
equation "d233 = FourthLayerCube"
equation "d234 = FourthLayerCube"
equation "d235 = SecondLayerSquare"
equation "d236 = SecondLayerSquare"
equation "d237 = SecondLayerIndent"
equation "d238 = SecondLayerSquare"
equation "d240 = SecondLayerIndent"
equation "d241 = SecondLayerSquare"
equation "d243 = SecondLayerIndent"
equation "d246 = SecondLayerSquare"
equation "d247 = SecondLayerSquare"
equation "d248 = SecondLayerIndent"
equation "d251 = SecondLayerIndent"
equation "d255 = SecondLayerIndent"
equation "d256 = SecondLayerSquare"
equation "d260 = SecondLayerIndent"
equation "d261 = SecondLayerIndent"
equation "d262 = SecondLayerIndent"
equation "d263 = SecondLayerIndent"
equation "d264 = SecondLayerSide"
equation "d265 = SecondLayerSide"
equation "d266 = SecondLayerSide"
equation "d267 = SecondLayerIndent"
equation "d268 = SecondLayerSide"
equation "d269 = FourthLayerDepth"
equation "d273 = SecondLayerDepth"
equation "d275 = ThirdLayerDepth"
equation "d284 = FirstLayerCube"
equation "d285 = FirstLayerCube"
equation "d286 = FirstLayerSquare"
equation "d287 = FirstLayerSquare"
equation "d293 = FirstLayerSquare"
equation "d294 = FirstLayerSquare"
equation "d297 = FirstLayerIndent"
equation "d298 = FirstLayerSquare"
equation "d299 = FirstLayerIndent"
equation "d300 = FirstLayerIndent"
equation "d301 = FirstLayerIndent"
equation "d302 = FirstLayerIndent"
equation "d303 = FirstLayerSide"
equation "d305 = FirstLayerSide"
equation "d306 = FirstLayerIndent"
equation "d307 = FirstLayerSide"
equation "d308 = FirstLayerSquare"
equation "d309 = FirstLayerSquare"
equation "d310 = FirstLayerSquare"
equation "d311 = FirstLayerSquare"
equation "d313 = FirstLayerSquare"
equation "d314 = FirstLayerSquare"
equation "d316 = FirstLayerSquare"
equation "d317 = FirstLayerSquare"
equation "d321 = FirstLayerSide"
equation "d322 = FirstLayerSide"
equation "d325 = SecondLayerSquare"
equation "d326 = SecondLayerSquare"
equation "d327 = SecondLayerSquare"
equation "d328 = SecondLayerSquare"
equation "d329 = SecondLayerSquare"
equation "d330 = SecondLayerSquare"
equation "d331 = SecondLayerSquare"
equation "d332 = SecondLayerSquare"
equation "d333 = SecondLayerSquare"
equation "d334 = SecondLayerSquare"
equation "d335 = SecondLayerSquare"
equation "d336 = FirstLayerSquare"
equation "d339 = FirstLayerSide"
equation "d340 = FirstLayerSquare"
equation "d341 = FirstLayerSquare"
equation "d342 = FirstLayerIndent"
equation "d343 = FirstLayerIndent"
equation "d344 = FirstLayerIndent"
equation "d345 = FirstLayerSquare"
equation "d346 = FirstLayerSquare"
equation "d348 = FirstLayerIndent"
equation "d349 = FirstLayerIndent"
equation "d350 = FirstLayerSide"
equation "d351 = FirstLayerSide"
equation "d352 = FirstLayerDepth"
named bodies: "FourthLayer", "ThirdLayer", "SecondLayer", "FirstLayer"
